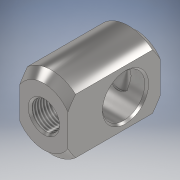
# Autodesk Inventor part: IMS-01-002
Saved by Autodesk Inventor 2021 (Build 250183000, 183)
## iProperties
Created: 2020-09-10
Part Number: IMS-01-002
Material: Steel, Carbon
Document SubType Name: Modeling
Designer: mahra
Density: 7.85 g/cm^3
Appearance: Semi-Polished
Mass: 208.743 g
Surface Area: 73.4427 cm^2
Volume: 26.5915 cm^3
Author: mahra
Autodesk Inventor part; units mm, degrees
ref_plane "YZ Plane" through (0, 0, 0) normal (1, 0, 0) x (0, 1, 0)
ref_plane "XZ Plane" through (0, 0, 0) normal (0, 1, 0) x (-1, 0, 0)
ref_plane "XY Plane" through (0, 0, 0) normal (0, 0, 1) x (1, 0, 0)
sketch "Sketch1" plane through (0, 0, 0) normal (0, 0, 1) x (1, 0, 0)
  circle A0 centre (0, 0) radius 19
  dimension "d0" = 38
  constraints: 1 centre point, 1 coincident
  measures "d0" diameter of A0
extrude "Extrusion1" add sketch "Sketch1" along normal blind 48
sketch "Sketch2" plane through (0, 0, 48) normal (0, 0, 1) x (1, 0, 0)
  line L0 (12.5, 21.9531) -> (30.6636, 21.9531)
  line L1 (30.6636, 21.9531) -> (30.6636, -19.8764)
  line L2 (30.6636, -19.8764) -> (12.5, -19.8764)
  line L3 (12.5, -19.8764) -> (12.5, 21.9531)
  point P0 (0, 0)
  dimension "d3" = 12.5
  constraints: 8 end point, 2 parallel, 1 horizontal, 1 perpendicular
  measures "d3" distance from line of point (0, 0) L3
extrude "Extrusion2" cut sketch "Sketch2" against normal through all
pattern_circular "Circular Pattern1" count 2 over 360 about axis through (0, 0, 0) along (0, 0, 1) of "Extrusion2"
sketch "Sketch3" plane through (12.5, -14.3091, 48) normal (1, 0, 0) x (0, 0, -1)
  circle A0 centre (30, 14.3091) radius 11
  line L0 (48, 28.6182) -> (48, 0) projected
  point P0 (48, 14.3091)
  point P1 (48, 14.3091)
  dimension "d9" = 22
  dimension "d10" = 18
  constraints: 1 centre point, 1 horizontal alignment, 1 midpoint
  measures "d9" diameter of A0
  measures "d10" distance from line of L0 A0.centre
extrude "Extrusion3" cut sketch "Sketch3" against normal through all
sketch "Sketch4" plane through (0, 0, 48) normal (0, 0, 1) x (1, 0, 0)
  arc A0 (12.5, 14.3091) -> (-12.5, 14.3091) centre (0, 0) ccw projected
  constraints: 1 coincident
hole "Hole1" at (0, 0, 48) direction (0, 0, -1) diameter 14.376 depth 39.3 tip angle 118 thread size "M16x1.5" class "6H" standard "ISO Metric profile"
chamfer "Chamfer1" distance 4 angle 45 4 edges at (0, 19, 0) (0, -19, 0) (0, 19, 48) (0, -19, 48)
chamfer "Chamfer2" distance 1 angle 45 1 edges at (0, 7.188, 48)
chamfer "Chamfer3" distance 1 angle 45 2 edges at (12.5, 0, 29) (-12.5, 0, 29)
body "Solid1"
